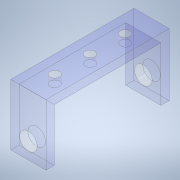
# Autodesk Inventor part: Papa John Bolt Plate
Saved by Autodesk Inventor 2020 (Build 240168000, 168)
## iProperties
Created: 2020-01-31
Part Number: Papa John Bolt Plate
Material: Polycarbonate, Clear
Document SubType Name: Modeling
Designer: aidan
Density: 1.2 g/cm^3
Appearance: Polycarbonate - Clear
Author: aidan
Autodesk Inventor part; units mm, degrees
ref_plane "YZ Plane" through (0, 0, 0) normal (1, 0, 0) x (0, 1, 0)
ref_plane "XZ Plane" through (0, 0, 0) normal (0, 1, 0) x (-1, 0, 0)
ref_plane "XY Plane" through (0, 0, 0) normal (0, 0, 1) x (1, 0, 0)
sketch "Sketch1" plane through (0, 0, 0) normal (1, 0, 0) x (0, 1, 0)
  line L0 (-1.2434, 22.2577) -> (20.8038, 22.2577)
  line L1 (20.8038, 22.2577) -> (20.8038, -15.9039)
  line L2 (17.8066, 19.2605) -> (-1.2434, 19.2605)
  line L3 (-1.2434, 19.2605) -> (-1.2434, 22.2577)
  line L4 (20.8038, 22.2577) -> (1.0601, 22.2577)
  line L5 (17.8066, 19.2605) -> (17.8066, -19.1951)
  line L6 (1.0601, -22.1923) -> (20.8038, -22.1923)
  line L7 (20.8038, -22.1923) -> (20.8038, 22.2577)
  line L8 (20.8038, -22.1923) -> (-1.7276, -22.1923)
  line L9 (-1.7276, -22.1923) -> (-1.7276, -19.1951)
  line L10 (-1.7276, -19.1951) -> (17.8066, -19.1951)
  line L11 (20.8038, -19.8757) -> (20.8038, -22.1923)
  point P0 (0, 0)
  dimension "d0" = 2.9972
  dimension "d1" = 19.05
  dimension "d2" = 44.45
  dimension "d3" = 2.9972
  constraints: 24 end point, 7 parallel, 3 horizontal, 3 perpendicular
  measures "d0" distance of L2.end L0.start
  measures "d1" distance of L2.start L2.end
  measures "d2" distance between parallel lines of L6 L0
  measures "d3" distance between parallel lines of L1 L5
extrude "Extrusion1" add sketch "Sketch1" along normal blind 12.7
sketch "Sketch2" plane through (0, -1.2434, 22.2577) normal (0, 0, 1) x (1, 0, 0)
  circle A0 centre (6.35, 5.8657) radius 3.175
  line L0 (0, -0.4843) -> (12.7, -0.4843) projected
  line L1 (12.7, 22.0472) -> (12.7, 0) projected
  point P0 (0, 1.2434)
  dimension "d6" = 6.35
  dimension "d7" = 6.35
  dimension "d8" = 6.35
  constraints: 1 centre point
  measures "d6" diameter of A0
  measures "d7" distance from line of L0 A0.centre
  measures "d8" distance from line of L1 A0.centre
extrude "Extrusion2" cut sketch "Sketch2" against normal through all
sketch "Sketch3" plane through (0, 20.8038, 22.2577) normal (0, 1, 0) x (1, 0, 0)
  line L0 (9.525, 0) -> (3.175, 0) projected
  line L1 (6.35, 0) -> (6.35, 44.45) construction
  line L2 (0, 44.45) -> (12.7, 44.45) projected
  circle A0 centre (6.35, 9.525) radius 1.7272
  circle A1 centre (6.35, 22.225) radius 1.7272
  circle A2 centre (6.35, 34.925) radius 1.7272
  point P0 (0, 22.2577)
  dimension "d11" = 3.4544
  dimension "d12" = 12.7
  dimension "d13" = 12.7
  constraints: 3 centre point, 3 midpoint, 2 end point, 2 equal radius, 2 point on line
  measures "d11" diameter of A2
  measures "d12" distance of A0.centre A1.centre
  measures "d13" distance of A2.centre A1.centre
hole "Hole1" at (6.35, 20.8038, -12.6673) at (6.35, 20.8038, 0.0327) at (6.35, 20.8038, 12.7327) direction (0, -1, 0) diameter 3.4544 end through all
body "Solid1"
